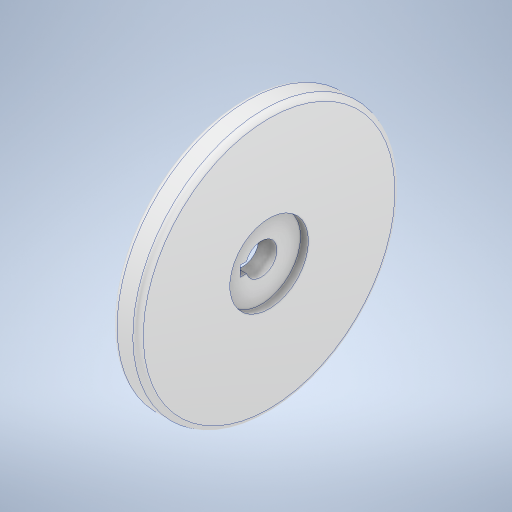
# Autodesk Inventor part: BRAKE DISC
Saved by Autodesk Inventor 2023 (Build 270158000, 158)
## iProperties
Created: 2022-08-21
Part Number: BRAKE DISC
Material: Aluminum 6061
Document SubType Name: Modeling
Designer: D.C. Eksteen
Density: 2.7 g/cm^3
Appearance: Aluminum - Flat
Mass: 209.831 g
Surface Area: 190.103 cm^2
Volume: 77.7152 cm^3
Author: D.C. Eksteen
Title: BRAKE DISC
Autodesk Inventor part; units mm, degrees
ref_plane "YZ Plane" through (0, 0, 0) normal (1, 0, 0) x (0, 1, 0)
ref_plane "XZ Plane" through (0, 0, 0) normal (0, 1, 0) x (-1, 0, 0)
ref_plane "XY Plane" through (0, 0, 0) normal (0, 0, 1) x (1, 0, 0)
sketch "Sketch1" plane through (0, 0, 0) normal (1, 0, 0) x (0, 1, 0)
  circle A0 centre (0, 0) radius 50
  dimension "d0" = 100
  constraints: 1 centre point, 1 coincident
  measures "d0" diameter of A0
extrude "Extrusion1" add sketch "Sketch1" along normal blind 10
sketch "Sketch2" plane through (10, 0, 0) normal (1, 0, 0) x (0, 0, -1)
  circle A0 centre (0, 0) radius 50 projected
hole "Hole1" at (10, 0, 0) direction (-1, 0, 0) diameter 12 depth 10
fillet "Fillet1" radius 2 2 edges at (0, -50, 0) (10, -50, 0)
sketch "Sketch4" plane through (10, 0, 0) normal (1, 0, 0) x (0, 0, -1)
  circle A0 centre (0, 0) radius 15
  dimension "d18" = 30
  constraints: 1 centre point, 1 coincident
  measures "d18" diameter of A0
extrude "Extrusion3" cut sketch "Sketch4" against normal blind 3
sketch "Sketch5" plane through (7, 0, 0) normal (1, 0, 0) x (0, 0, -1)
  circle A0 centre (0, 0) radius 6 projected
  line L0 (-6, 0) -> (-6, 2)
  line L1 (-6, 2) -> (-8, 2)
  line L2 (-8, 2) -> (-8, -2)
  line L3 (-8, -2) -> (-6, -2)
  line L4 (-6, -2) -> (-6, 0)
  line L5 (-6, -2) -> (-4.5, -2)
  line L6 (-4.5, -2) -> (-4.5, 2)
  line L7 (-4.5, 2) -> (-6, 2)
  point P0 (-7, -2)
  dimension "d21" = 2
  dimension "d22" = 4
  dimension "d23" = 2
  dimension "d24" = 1.5
  dimension "d25" = 4
  constraints: 16 end point, 5 perpendicular, 3 vertical, 1 horizontal, 1 horizontal alignment, 1 midpoint, 1 point on line, 1 other
  measures "d21" distance between parallel lines of L4 L2
  measures "d22" distance from line of L1 point (-7, -2)
  measures "d23" distance from line of L0.start L3
  measures "d24" distance of L3.end L5.end
  measures "d25" distance of L5.end L6.end
extrude "Extrusion4" cut sketch "Sketch5" against normal blind 7 contours L7 L6 L5 A0 | A0 L0 L7 | L5 L4 A0 | L4 L3 L2 L1 L0 picked at (-5, 0)
body "Solid1"
